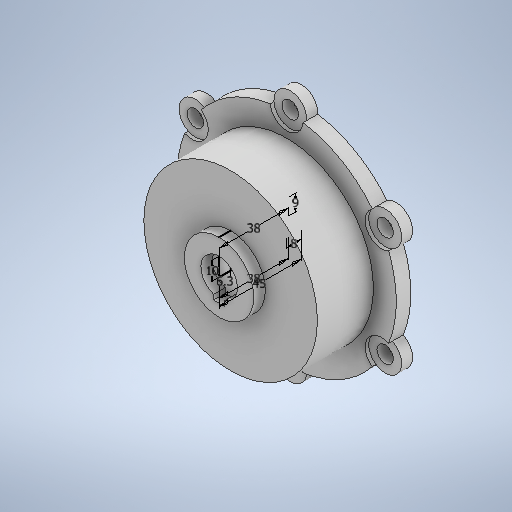
# Autodesk Inventor part: Bai13
Saved by Autodesk Inventor 2025.1 (Build 291241000, 241)
## iProperties
Created: 2024-10-02
Part Number: Bai13
Material: Generic
Document SubType Name: Modeling
Designer: msi
Density: 1 g/cm^3
Appearance: Default
Author: msi
Autodesk Inventor part; units mm, degrees
ref_plane "YZ Plane" through (0, 0, 0) normal (1, 0, 0) x (0, 1, 0)
ref_plane "XZ Plane" through (0, 0, 0) normal (0, 1, 0) x (-1, 0, 0)
ref_plane "XY Plane" through (0, 0, 0) normal (0, 0, 1) x (1, 0, 0)
sketch "Sketch1" plane through (0, 0, 0) normal (0, 0, 1) x (1, 0, 0)
  circle A0 centre (0, 0) radius 19
  circle A1 centre (0, 0) radius 10
  line L0 (0, -10) -> (0, -12.3)
  line L1 (0, -12.3) -> (-3, -12.3)
  line L2 (0, -12.3) -> (3, -12.3)
  line L3 (3, -12.3) -> (3, -9.5394)
  line L4 (-3, -12.3) -> (-3, -9.5394)
  circle A2 centre (0, 0) radius 66
  circle A3 centre (0, 0) radius 60
  circle A4 centre (0, 0) radius 47.5
  circle A5 centre (0, 60) radius 4.5
  circle A6 centre (-51.9615, 30) radius 4.5
  circle A7 centre (-51.9615, -30) radius 4.5
  circle A8 centre (0, -60) radius 4.5
  circle A9 centre (51.9615, -30) radius 4.5
  circle A10 centre (51.9615, 30) radius 4.5
  circle A11 centre (0, 60) radius 9
  circle A12 centre (-51.9615, 30) radius 9
  circle A13 centre (-51.9615, -30) radius 9
  circle A14 centre (0, -60) radius 9
  circle A15 centre (51.9615, -30) radius 9
  circle A16 centre (51.9615, 30) radius 9
  point P0 (-7.0256, 65.625)
  point P1 (-53.3201, 38.8969)
  point P2 (-60.3457, 26.7281)
  point P3 (-7.0256, -65.625)
  point P4 (7.0256, -65.625)
  point P5 (53.3201, -38.8969)
  point P6 (60.3457, -26.7281)
  point P7 (7.0256, 65.625)
  point P8 (55.8643, 21.8902)
  point P9 (46.8896, 37.4348)
  point P10 (8.9747, 59.325)
  point P11 (-8.9747, 59.325)
  point P12 (-46.8896, 37.4348)
  point P13 (-55.8643, 21.8902)
  point P14 (-55.8643, -21.8902)
  point P15 (-46.8896, -37.4348)
  point P16 (-8.9747, -59.325)
  point P17 (8.9747, -59.325)
  point P18 (46.8896, -37.4348)
  point P19 (55.8643, -21.8902)
  dimension "d6" = 120
  dimension "d0" = 38
  dimension "d1" = 20
  dimension "d2" = 2.3
  dimension "d3" = 3
  dimension "d4" = 3
  dimension "d5" = 132
  dimension "d7" = 95
  dimension "d8" = 9
  dimension "d11" = 360
  dimension "d13" = 18
  dimension "d16" = 360
  constraints: 16 centre point, 10 end point, 6 coincident, 3 point on circle, 2 horizontal, 2 vertical, 1 perpendicular, 29 other
  measures "d0" diameter of A0
  measures "d1" diameter of A1
  measures "d2" distance of L0.start L0.end
  measures "d3" distance of L0.end L1.end
  measures "d4" distance of L0.end L2.end
  measures "d5" diameter of A2
  measures "d7" diameter of A4
  measures "d8" diameter of A5
  measures "d13" diameter of A11
sketch "Sketch2" plane through (0, 0, 0) normal (1, 0, 0) x (0, 1, 0)
  line L0 (0, 0) -> (0, -45)
  line L1 (0, 0) -> (0, -38)
  line L2 (0, -45) -> (0, -37)
  line L3 (0, 0) -> (10, 0)
  line L4 (10, 0) -> (10, -38)
  line L5 (10, -38) -> (19, -38)
  line L6 (19, 0) -> (19, -38)
  line L7 (0, 0) -> (0, -6.3)
  line L8 (0, -6.3) -> (19, -6.3)
  dimension "d18" = 45
  dimension "d19" = 38
  dimension "d20" = 8
  dimension "d21" = 10
  dimension "d22" = 38
  dimension "d23" = 9
  dimension "d34" = 6.3
  constraints: 18 end point, 4 point on line, 3 perpendicular, 2 vertical, 1 horizontal
  measures "d18" distance of L0.start L0.end
  measures "d19" distance of L0.start L1.end
  measures "d20" distance of L0.end L2.end
  measures "d21" distance of L0.start L3.end
  measures "d22" distance of L3.end L4.end
  measures "d23" distance of L4.end L5.end
  measures "d34" distance of L0.start L7.end
extrude "Extrusion3" add sketch "Sketch1" against normal blind 6.3 contours A0
extrude "Extrusion4" add sketch "Sketch1" against normal blind 37 contours A4
extrude "Extrusion5" cut sketch "Sketch1" against normal blind 6.3 contours A4
extrude "Extrusion6" add sketch "Sketch1" against normal blind 45 contours A3 A15 A14 A13 A12 A11 A16
extrude "Extrusion8" cut sketch "Sketch1" against normal blind 37 contours A3 A15 A14 A13 A12 A11 A16
extrude "Extrusion9" add sketch "Sketch1" against normal blind 45 contours A16 A3 A10 A2 | A2 A16 | A15 A2 | A2 A15 A3 A9 | A16 A3 A10 | A3 A9 A15 | A11 A3 A5 A2 | A2 A11 | A10 A3 | A3 A10 | A14 A2 | A2 A14 A3 A8 | A9 A3 | A3 A9 | A11 A3 A5 | A3 A8 A14 | A12 A3 A6 A2 | A2 A12 | A5 A3 | A3 A5 | A13 A2 | A2 A13 A3 A7 | A8 A3 | A3 A8 | A12 A3 A6 | A3 A7 A13 | A6 A3 | A3 A6 | A7 A3 | A3 A7
extrude "Extrusion10" cut sketch "Sketch1" against normal blind 39 contours A16 A3 A10 A2 | A2 A16 | A15 A2 | A2 A15 A3 A9 | A16 A3 A10 | A3 A9 A15 | A11 A3 A5 A2 | A2 A11 | A10 A3 | A3 A10 | A14 A2 | A2 A14 A3 A8 | A9 A3 | A3 A9 | A11 A3 A5 | A3 A8 A14 | A12 A3 A6 A2 | A2 A12 | A5 A3 | A3 A5 | A13 A2 | A2 A13 A3 A7 | A8 A3 | A3 A8 | A12 A3 A6 | A3 A7 A13 | A6 A3 | A3 A6 | A7 A3 | A3 A7
extrude "Extrusion11" cut sketch "Sketch1" against normal blind 45 contours A10 A3 | A3 A10 | A9 A3 | A3 A9 | A5 A3 | A3 A5 | A8 A3 | A3 A8 | A6 A3 | A3 A6 | A7 A3 | A3 A7
body "Solid2"
